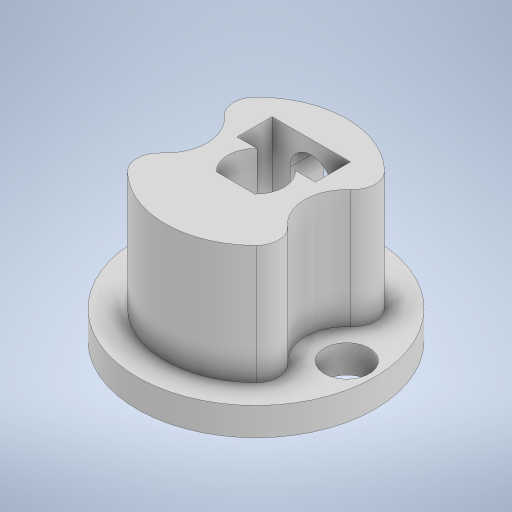
# Autodesk Inventor part: acople
Saved by Autodesk Inventor 2024 (Build 280153000, 153)
## iProperties
Created: 2024-08-09
Part Number: acople
Material: Generic
Document SubType Name: Modeling
Designer: David Ricaurte
Density: 1 g/cm^3
Appearance: Default
Author: David Ricaurte
Autodesk Inventor part; units mm, degrees
ref_plane "YZ Plane" through (0, 0, 0) normal (1, 0, 0) x (0, 1, 0)
ref_plane "XZ Plane" through (0, 0, 0) normal (0, 1, 0) x (-1, 0, 0)
sketch "Sketch1" plane through (0, 0, 0) normal (0, 1, 0) x (-1, 0, 0)
  circle A0 centre (0, 0) radius 4.5
  circle A1 centre (0, 0) radius 2
  circle A2 centre (0, 0) radius 1.45
  line L0 (0, -1.45) -> (1.3775, -1.45)
  line L1 (0, -1.45) -> (-1.3775, -1.45)
  line L2 (0, 1.45) -> (-1.3775, 1.45)
  line L3 (0, 1.45) -> (1.3775, 1.45)
  dimension "d0" = 9
  dimension "d1" = 4
  dimension "d2" = 2.9
  constraints: 8 end point, 6 point on circle, 3 centre point, 3 coincident, 2 point on line, 2 tangent, 1 horizontal, 1 parallel
  measures "d0" diameter of A0
  measures "d1" diameter of A1
  measures "d2" diameter of A2
extrude "Extrusion1" add sketch "Sketch1" along normal blind 7 contours A0 | L3 L2 A1 | A1 L1 L0
sketch "Sketch2" plane through (0, 7, 0) normal (0, 1, 0) x (1, 0, 0)
  line L0 (-1.3775, 1.45) -> (1.3775, 1.45) projected
  line L1 (0, 1.45) -> (0, 3.85)
  line L2 (1.3775, -0.95) -> (-1.3775, -0.95)
  line L3 (-1.3775, -0.95) -> (-1.3775, 3.85)
  line L4 (-1.3775, 3.85) -> (1.3775, 3.85)
  line L5 (1.3775, 3.85) -> (1.3775, -0.95)
  line L6 (1.3775, -0.95) -> (-1.3775, 3.85) construction
  line L7 (-1.3775, -0.95) -> (1.3775, 3.85) construction
  line L8 (2.75, -0.95) -> (-2.75, -0.95)
  line L9 (-2.75, -0.95) -> (-2.75, 3.85)
  line L10 (-2.75, 3.85) -> (2.75, 3.85)
  line L11 (2.75, 3.85) -> (2.75, -0.95)
  line L12 (2.75, -0.95) -> (-2.75, 3.85) construction
  line L13 (-2.75, -0.95) -> (2.75, 3.85) construction
  circle A0 centre (0, 0) radius 6.5
  circle A1 centre (0, 0) radius 4.5
  dimension "d5" = 2.4
  dimension "d6" = 5.5
  dimension "d7" = 13
  constraints: 26 end point, 5 midpoint, 4 parallel, 2 centre point, 2 coincident, 2 horizontal, 2 perpendicular, 1 point on line, 1 vertical
  measures "d5" distance of L1.start L1.end
  measures "d6" distance of L9.end L10.end
  measures "d7" diameter of A0
extrude "Extrusion2" add sketch "Sketch2" against normal blind 7 contours A1 L9 L10 | L10 L11 A1 | A0
sketch "Sketch3" plane through (0, 7, 0) normal (0, 1, 0) x (1, 0, 0)
  line L0 (-1.3775, 1.45) -> (1.3775, 1.45) projected
  line L1 (0, 1.45) -> (0, 3.95)
  line L2 (2.8, -1.05) -> (-2.8, -1.05)
  line L3 (-2.8, -1.05) -> (-2.8, 3.95)
  line L4 (-2.8, 3.95) -> (2.8, 3.95)
  line L5 (2.8, 3.95) -> (2.8, -1.05)
  line L6 (2.8, -1.05) -> (-2.8, 3.95) construction
  line L7 (-2.8, -1.05) -> (2.8, 3.95) construction
  line L8 (0, 1.45) -> (-2.8, 1.45)
  line L9 (0, 1.45) -> (2.8, 1.45)
  point P0 (0, 0)
  dimension "d10" = 2.5
  dimension "d11" = 5.6
  constraints: 18 end point, 5 midpoint, 2 parallel, 1 horizontal, 1 perpendicular, 1 vertical
  measures "d10" distance of L1.start L1.end
  measures "d11" distance of L3.end L4.end
extrude "Extrusion3" cut sketch "Sketch3" against normal blind 7 contours L8 L3 L4 L1 L0 | L1 L4 L5 L9 L0
ref_plane "Work Plane1" through (-2.8, 7, -8.95) normal (0, 0, 1) x (1, 0, 0)
sketch "Sketch5" plane through (-2.8, 7, -8.95) normal (0, 0, 1) x (1, 0, 0)
  circle A0 centre (2.8, -2.4541) radius 1.5
  line L0 (2.8, -2.4541) -> (2.8, -7)
  circle A1 centre (2.8, -3.9541) radius 1.5
  circle A2 centre (2.8, -4.8651) radius 1.5
  line L1 (1.3, -4.8651) -> (1.3, -2.4541)
  line L2 (4.3, -4.8651) -> (4.3, -2.4541)
  point P0 (4.3, -4.8651)
  dimension "d17" = 3
  dimension "d15" = 3
  dimension "d16" = 3
  constraints: 6 end point, 2 centre point, 2 point on circle, 2 point on line, 2 symmetric about line, 2 vertical, 1 parallel, 3 other
  measures "d15" diameter of A0
  measures "d16" diameter of A1
extrude "Extrusion4" cut sketch "Sketch5" along normal blind 6
sketch "Sketch6" plane through (0, 0, 0) normal (0, -1, 0) x (1, 0, 0)
  circle A0 centre (0, 0) radius 6.5
  constraints: 1 centre point, 1 coincident
extrude "Extrusion5" add sketch "Sketch6" along normal blind 1.5
sketch "Sketch7" plane through (0, -1.5, 0) normal (0, -1, 0) x (1, 0, 0)
  line L0 (-3.5, -3.5) -> (3.5, -3.5)
  line L1 (3.5, -3.5) -> (3.5, 3.5)
  line L2 (3.5, 3.5) -> (-3.5, 3.5)
  line L3 (-3.5, 3.5) -> (-3.5, -3.5)
  line L4 (-3.5, -3.5) -> (3.5, 3.5) construction
  line L5 (3.5, -3.5) -> (-3.5, 3.5) construction
  point P0 (0, 0)
  dimension "d22" = 7
  dimension "d23" = 7
  constraints: 12 end point, 2 midpoint, 2 parallel, 1 horizontal, 1 perpendicular
  measures "d22" distance of L2.end L1.end
  measures "d23" distance of L1.end L0.end
extrude "Extrusion6" add sketch "Sketch7" along normal blind 6
sketch "Sketch8" plane through (0, -1.5, 0) normal (0, -1, 0) x (1, 0, 0)
  arc A0 (-1.3775, 1.45) -> (-1.3775, -1.45) centre (0, 0) ccw projected
  circle A1 centre (0, 0) radius 8.6758
  constraints: 1 centre point, 1 coincident
extrude "Extrusion7" cut sketch "Sketch8" along normal blind 10
sketch "Sketch9" plane through (0, -1.5, 0) normal (0, -1, 0) x (1, 0, 0)
  point P0 (0, 0)
sketch "Sketch10" plane through (0, -1.5, 0) normal (0, -1, 0) x (1, 0, 0)
  circle A0 centre (0, 0) radius 6.5
  circle A1 centre (6.5, 0) radius 3
  circle A2 centre (-6.5, 0) radius 3
  dimension "d28" = 13
  dimension "d29" = 6
  dimension "d30" = 6
  constraints: 3 centre point, 2 point on circle, 1 coincident
  measures "d28" diameter of A0
  measures "d29" diameter of A1
  measures "d30" diameter of A2
extrude "Extrusion8" cut sketch "Sketch10" against normal through all contours A0 A1 | A0 A1 | A2 A0 | A0 A2
sketch "Sketch11" plane through (0, -1.5, 0) normal (0, -1, 0) x (1, 0, 0)
  circle A0 centre (0, 0) radius 8.5
  dimension "d33" = 17
  constraints: 1 centre point, 1 coincident
  measures "d33" diameter of A0
extrude "Extrusion9" add sketch "Sketch11" along normal blind 2
sketch "Sketch12" plane through (0, -3.5, 0) normal (0, -1, 0) x (1, 0, 0)
  arc A0 (1.3775, -1.45) -> (1.3775, 1.45) centre (0, 0) ccw projected
  circle A1 centre (0, 0) radius 6.5
  arc A2 (-5.8077, -2.919) -> (-5.8077, 2.919) centre (-6.5, 0) ccw projected
  circle A3 centre (-6.5, 0) radius 1.6
  circle A4 centre (6.5, 0) radius 1.6
  dimension "d36" = 13
  dimension "d37" = 3.2
  dimension "d38" = 3.2
  constraints: 3 centre point, 2 coincident, 1 point on circle
  measures "d36" diameter of A1
  measures "d37" diameter of A3
  measures "d38" diameter of A4
extrude "Extrusion10" cut sketch "Sketch12" against normal through all contours A1 A4 | A1 A4 | A3 A1 | A1 A3
fillet "Fillet1" radius 1.6 4 edges at (5.8077, 2.75, 2.919) (5.8077, 2.75, -2.919) (-5.8077, 2.75, 2.919) (-5.8077, 2.75, -2.919)
body "Solid1"
